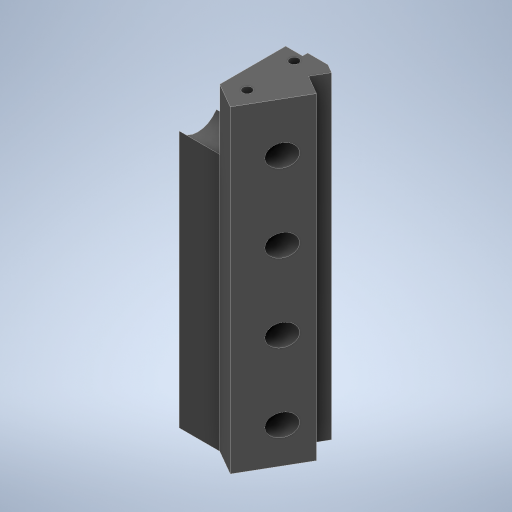
# Autodesk Inventor part: rail_base_outside
Saved by Autodesk Inventor 2024.1 (Build 281209000, 209)
## iProperties
Created: 2025-01-17
Part Number: rail_base_outside
Material: 一般
Document SubType Name: Modeling
Designer: hibik
Density: 1 g/cm^3
Appearance: 既定
Author: hibik
Autodesk Inventor part; units mm, degrees
sketch "スケッチ1" plane through (0, 0, 0) normal (0, 1, 0) x (-1, 0, 0)
  line L0 (0, 0) -> (-19.196896, -33.25)
  line L1 (0, 0) -> (30, 0) construction
  line L2 (30, 0) -> (30, -18)
  line L3 (30, -18) -> (18.452995, -38)
  line L4 (18.452995, -38) -> (-10.969655, -38)
  line L5 (-10.969655, -38) -> (-19.196896, -33.25)
  line L6 (30, -1.5) -> (-0.866025, -1.5)
  line L7 (25, -1.5) -> (5, -1.5)
  line L8 (5, -1.5) -> (5, -8)
  line L9 (5, -8) -> (25, -8) construction
  line L10 (25, -8) -> (25, -1.5)
  line L11 (30, -18) -> (21.919873, -13.334936)
  line L12 (21.919873, -13.334936) -> (25, -8)
  line L13 (30, -10.5) -> (25.669873, -8) construction
  line L14 (25.669873, -8) -> (22.422278, -13.625) construction
  line L15 (22.422278, -13.625) -> (26.752405, -16.125) construction
  line L16 (26.752405, -16.125) -> (30, -10.5) construction
  line L17 (5, -8) -> (12, -8)
  line L18 (12, -8) -> (12, -17)
  line L19 (12, -17) -> (5, -17)
  line L20 (5, -17) -> (5, -8) construction
  line L21 (5, -17) -> (0, -17)
  line L22 (0, -17) -> (-7.361216, -12.75)
  line L23 (0, -38) -> (0, -28)
  line L24 (0, -28) -> (24.226497, -28)
  line L25 (-13.567731, -36.5) -> (-11.067731, -32.169873)
  line L26 (-11.067731, -32.169873) -> (-16.696896, -28.919873)
  line L27 (0, -38) -> (-5, -38)
  line L28 (-5, -38) -> (-5, -36.5)
  line L29 (-5, -36.5) -> (0, -36.5)
  line L30 (0, -36.5) -> (0, -38)
  point P0 (-5, -38)
  point P1 (0, -36.5)
  dimension "d0" = 60
  dimension "d1" = 30
  dimension "d4" = 9.5
  dimension "d5" = 1.5
  dimension "d6" = 5
  dimension "d7" = 5
  dimension "d8" = 6.5
  dimension "d10" = 5
  dimension "d12" = 6.16025
  dimension "d14" = 9
  dimension "d15" = 7
  dimension "d18" = 10
  dimension "d19" = 10
  dimension "d20" = 6.5
  dimension "d21" = 5
  dimension "d22" = 3
  dimension "d23" = 5
  dimension "d24" = 1.5
  dimension "d26" = 38
  dimension "d27" = 18
  constraints: 62 end point, 11 parallel, 10 perpendicular, 10 point on line, 6 horizontal, 2 collinear, 2 vertical, 1 midpoint, 1 vertical alignment
  measures "d0" angle of L1 L0
  measures "d1" distance of L0.start L1.end
  measures "d4" distance from line of L4.end L0
  measures "d5" distance between parallel lines of L1 L6
  measures "d6" distance between parallel lines of L2 L10
  measures "d7" distance from line of L0.start L8
  measures "d8" distance of L9.end L7.start
  measures "d10" distance between parallel lines of L14 L16
  measures "d12" distance from line of L11 L9.end
  measures "d14" distance of L17.end L18.end
  measures "d15" distance of L18.end L19.end
  measures "d18" distance between parallel lines of L4 L24
  measures "d19" distance from line of L2.end L24
  measures "d20" distance between parallel lines of L0 L25
  measures "d21" distance between parallel lines of L5 L26
  measures "d22" distance from line of L4.end L25
  measures "d23" distance of L28.end L29.end
  measures "d24" distance of L27.end L28.end
  measures "d26" distance between parallel lines of L1 L4
  measures "d27" distance from line of L1 L2.end
extrude "押し出し1" add sketch "スケッチ1" along normal blind 94 contours L22 L21 L19 L18 L17 L8 L6 L10 L12 L11 L3 L24 L23 L29 L28 L4 L5 L25 L26 L0
sketch "スケッチ3" plane through (-12, 0, -8) normal (1, 0, 0) x (0, 0, -1)
  circle A0 centre (14.5, 79.5) radius 5.5
  line L0 (9, 0) -> (9, 94)
  line L1 (20, 0) -> (20, 94)
  line L2 (0, 94) -> (9, 94)
  line L3 (0, 94) -> (-6.5, 94)
  line L4 (-6.5, 94) -> (0, 94)
  line L5 (0, 94) -> (9, 94)
  line L6 (9, 94) -> (4.75, 94)
  line L7 (4.75, 94) -> (20.919873, 94)
  line L8 (20.919873, 94) -> (24.169873, 94)
  line L9 (24.169873, 94) -> (28.5, 94)
  line L10 (28.5, 94) -> (30, 94)
  line L11 (30, 94) -> (28.5, 94)
  line L12 (28.5, 94) -> (20, 94)
  line L13 (20, 94) -> (10, 94)
  line L14 (10, 94) -> (5.334936, 94)
  line L15 (5.334936, 94) -> (0, 94)
  circle A1 centre (14.5, 79.5) radius 6.5
  point P0 (-8, 0)
  point P1 (9, 79.5)
  point P2 (20, 79.5)
  point P3 (9, 82.964102)
  point P4 (20, 82.964102)
  dimension "d28" = 11
  dimension "d29" = 14.5
  dimension "d32" = 13
  constraints: 2 centre point, 2 tangent, 1 coincident
  measures "d28" diameter of A0
  measures "d29" distance from line of L2 A0.centre
  measures "d32" diameter of A1
extrude "押し出し2" cut sketch "スケッチ3" along normal up to surface (12 mm away)
sketch "スケッチ4" plane through (-12, 0, -8) normal (1, 0, 0) x (0, 0, -1)
  arc A0 (9, 76.035898) -> (20, 76.035898) centre (14.5, 79.5) ccw
  circle A1 centre (14.5, 79.5) radius 1.6
  point P0 (-8, 0)
  dimension "d33" = 3.2
  constraints: 1 centre point, 1 coincident
  measures "d33" diameter of A1
extrude "押し出し3" cut sketch "スケッチ4" against normal blind 8
sketch "スケッチ5" plane through (0, 0, -36.5) normal (-1, 0, 0) x (0, 0, 1)
  circle A0 centre (14, 79.5) radius 1.6 construction
  circle A1 centre (14, 79.5) radius 1.6
  line L0 (0, 0) -> (0, 94) projected
  circle A2 centre (14, 56.5) radius 1.6
  circle A3 centre (14, 33.5) radius 1.6
  circle A4 centre (14, 10.5) radius 1.6
  point P0 (36.5, 0)
  dimension "d36" = 3.2
  dimension "d39" = 23
  constraints: 4 centre point, 1 coincident, 1 vertical, 6 other
  measures "d36" diameter of A1
  measures "d39" distance of A1.centre A2.centre
extrude "押し出し4" cut sketch "スケッチ5" along normal through all both and the other way through all
ref_plane "作業平面1" through (-15, 0, -8) normal (1, 0, 0) x (0, 0, -1)
sketch "スケッチ6" plane through (-15, 0, -8) normal (1, 0, 0) x (0, 0, -1)
  circle A0 centre (14.5, 56.5) radius 1.6
  circle A1 centre (14.5, 33.5) radius 1.6
  circle A2 centre (14.5, 10.5) radius 1.6
  line L0 (17.790897, 79.5) -> (16.145448, 76.65)
  line L1 (16.145448, 76.65) -> (12.854552, 76.65)
  line L2 (12.854552, 76.65) -> (11.209103, 79.5)
  line L3 (11.209103, 79.5) -> (12.854552, 82.35)
  line L4 (12.854552, 82.35) -> (16.145448, 82.35)
  line L5 (16.145448, 82.35) -> (17.790897, 79.5)
  line L6 (17.790897, 56.5) -> (16.145448, 53.65)
  line L7 (16.145448, 53.65) -> (12.854552, 53.65)
  line L8 (12.854552, 53.65) -> (11.209103, 56.5)
  line L9 (11.209103, 56.5) -> (12.854552, 59.35)
  line L10 (12.854552, 59.35) -> (16.145448, 59.35)
  line L11 (16.145448, 59.35) -> (17.790897, 56.5)
  line L12 (17.790897, 33.5) -> (16.145448, 30.65)
  line L13 (16.145448, 30.65) -> (12.854552, 30.65)
  line L14 (12.854552, 30.65) -> (11.209103, 33.5)
  line L15 (11.209103, 33.5) -> (12.854552, 36.35)
  line L16 (12.854552, 36.35) -> (16.145448, 36.35)
  line L17 (16.145448, 36.35) -> (17.790897, 33.5)
  line L18 (17.790897, 10.5) -> (16.145448, 7.65)
  line L19 (16.145448, 7.65) -> (12.854552, 7.65)
  line L20 (12.854552, 7.65) -> (11.209103, 10.5)
  line L21 (11.209103, 10.5) -> (12.854552, 13.35)
  line L22 (12.854552, 13.35) -> (16.145448, 13.35)
  line L23 (16.145448, 13.35) -> (17.790897, 10.5)
  circle A3 centre (14.5, 79.5) radius 1.6
  point P0 (-8, 0)
  dimension "d47" = 5.7
  constraints: 48 end point, 4 coincident, 4 horizontal, 3 parallel, 52 other
  measures "d47" distance between parallel lines of L1 L4
extrude "押し出し5" cut sketch "スケッチ6" against normal through all contours A0 | A1 | A2 | L0 L1 L2 L3 L4 L5 | L6 L7 L8 L9 L10 L11 | L12 L13 L14 L15 L16 L17 | L18 L19 L20 L21 L22 L23 | A3
ref_plane "作業平面2" through (2, 0, -36.5) normal (-1, 0, 0) x (0, 0, 1)
sketch "スケッチ7" plane through (2, 0, -36.5) normal (-1, 0, 0) x (0, 0, 1)
  circle A0 centre (14, 79.5) radius 1.6 projected
  circle A1 centre (14, 56.5) radius 1.6 projected
  circle A2 centre (14, 33.5) radius 1.6 projected
  circle A3 centre (14, 10.5) radius 1.6 projected
  circle A4 centre (14, 79.5) radius 3.25
  circle A5 centre (14, 56.5) radius 1.6 projected
  circle A6 centre (14, 56.5) radius 3.25
  circle A7 centre (14, 33.5) radius 3.25
  circle A8 centre (14, 10.5) radius 3.25
  point P0 (36.5, 0)
  dimension "d51" = 6.5
  dimension "d52" = 6.5
  dimension "d53" = 6.5
  dimension "d54" = 6.5
  constraints: 4 centre point, 4 coincident
  measures "d51" diameter of A4
  measures "d52" diameter of A6
  measures "d53" diameter of A7
  measures "d54" diameter of A8
extrude "押し出し6" cut sketch "スケッチ7" against normal through all contours A0 | A1 | A2 | A3 | A4 | A6 | A7 | A8
sketch "スケッチ8" plane through (-25, 0, -1.5) normal (0, 0, 1) x (1, 0, 0)
  circle A0 centre (5, 77) radius 1.6 construction
  circle A1 centre (15, 77) radius 1.6 construction
  circle A2 centre (5, 47) radius 1.6 construction
  circle A3 centre (15, 47) radius 1.6 construction
  circle A4 centre (5, 17) radius 1.6 construction
  circle A5 centre (15, 17) radius 1.6 construction
  circle A6 centre (5, 77) radius 1.35
  circle A7 centre (15, 77) radius 1.35
  circle A8 centre (5, 47) radius 1.35
  circle A9 centre (15, 47) radius 1.35
  circle A10 centre (5, 17) radius 1.35
  circle A11 centre (15, 17) radius 1.35
  point P0 (25, 0)
  dimension "d59" = 2.7
  constraints: 6 centre point, 6 coincident, 5 equal radius
  measures "d59" diameter of A6
extrude "押し出し7" cut sketch "スケッチ8" against normal blind 5
ref_plane "作業平面3" through (0, 7, 0) normal (0, -1, 0) x (1, 0, 0)
sketch "スケッチ9" plane through (0, 7, 0) normal (0, -1, 0) x (1, 0, 0)
  line L0 (0, -38) -> (10.1, -38)
  line L1 (10.1, -38) -> (10.1, -30.8)
  line L2 (10.1, -30.8) -> (0, -30.8)
  line L3 (0, -30.8) -> (0, -38)
  line L4 (10.969655, -38) -> (-1, -38)
  point P0 (0, 0)
  point P1 (0, -36.5)
  dimension "d61" = 10.1
  dimension "d62" = 7.2
  constraints: 8 end point, 2 parallel, 1 collinear, 1 horizontal, 1 perpendicular, 1 point on line
  measures "d61" distance of L2.end L1.end
  measures "d62" distance of L1.end L0.end
extrude "押し出し8" cut sketch "スケッチ9" against normal blind 7.2
sketch "スケッチ11" plane through (0, 7, 0) normal (0, 1, 0) x (1, 0, 0)
  line L0 (5, 36.5) -> (5, 38) projected
  line L1 (5, 38) -> (0, 38)
  line L2 (0, 38) -> (0, 36.5)
  line L3 (0, 36.5) -> (5, 36.5)
  line L4 (5, 36.5) -> (5, 38)
  point P0 (0, 0)
  constraints: 8 end point, 2 parallel, 1 horizontal, 1 perpendicular
extrude "押し出し9" add sketch "スケッチ11" against normal up to surface (7 mm away)
sketch "スケッチ12" plane through (0, 14.2, 0) normal (0, -1, 0) x (1, 0, 0)
  line L0 (5, -36.5) -> (0, -36.5) projected
  line L1 (5, -38) -> (0, -38)
  line L2 (0, -38) -> (0, -36.5)
  line L3 (0, -36.5) -> (5, -36.5)
  line L4 (5, -36.5) -> (5, -38)
  point P0 (0, 0)
  constraints: 8 end point, 2 parallel, 1 horizontal, 1 perpendicular
extrude "押し出し10" add sketch "スケッチ12" against normal blind 10
sketch "スケッチ14" plane through (0, 0, 0) normal (0, -1, 0) x (1, 0, 0)
  circle A0 centre (5, -34) radius 1.6 projected
  point P0 (0, 0)
extrude "押し出し11" cut sketch "スケッチ14" against normal blind 30
sketch "スケッチ15" plane through (0, 0, 0) normal (0, -1, 0) x (1, 0, 0)
  circle A0 centre (5, -34) radius 1.6 projected
  circle A1 centre (5, -34) radius 2.5
  point P0 (0, 0)
  dimension "d71" = 5
  constraints: 1 centre point, 1 coincident
  measures "d71" diameter of A1
extrude "押し出し12" cut sketch "スケッチ15" against normal blind 4 contours A0 | A1
sketch "スケッチ16" plane through (0, 24.2, 0) normal (0, 1, 0) x (1, 0, 0)
  circle A0 centre (5, 34) radius 1.6
  line L0 (3.354552, 36.85) -> (6.645448, 36.85)
  line L1 (6.645448, 36.85) -> (8.290897, 34)
  line L2 (8.290897, 34) -> (6.645448, 31.15)
  line L3 (6.645448, 31.15) -> (3.354552, 31.15)
  line L4 (3.354552, 31.15) -> (1.709103, 34)
  line L5 (1.709103, 34) -> (3.354552, 36.85)
  line L6 (8.290897, 34) -> (8.290897, 38)
  line L7 (1.709103, 34) -> (1.709103, 38)
  line L8 (8.290897, 38) -> (1.709103, 38)
  line L9 (5, 38) -> (0, 38)
  point P0 (0, 0)
  dimension "d74" = 5.7
  constraints: 18 end point, 2 horizontal, 2 vertical, 1 coincident, 1 collinear, 13 other
  measures "d74" distance between parallel lines of L3 L0
extrude "押し出し13" cut sketch "スケッチ16" against normal blind 4 contours A0 | L5 L7 L8 L6 L1 L0 | L0 L1 L2 L3 L4 L5
ref_plane "作業平面4" through (0, 14, 0) normal (0, -1, 0) x (1, 0, 0)
sketch "スケッチ17" plane through (0, 14, 0) normal (0, -1, 0) x (1, 0, 0)
  line L0 (-28.351924, -20.854552) -> (-29.301924, -19.209103)
  line L1 (-29.301924, -19.209103) -> (-28.351924, -20.854552)
  line L2 (-28.351924, -20.854552) -> (-26.451924, -24.145448)
  line L3 (-26.451924, -24.145448) -> (-25.501924, -25.790897)
  line L4 (-25.501924, -25.790897) -> (-26.451924, -24.145448)
  line L5 (-26.451924, -24.145448) -> (-28.351924, -20.854552)
  line L6 (-28.351924, -20.854552) -> (-29.301924, -19.209103)
  line L7 (-29.301924, -19.209103) -> (-28.351924, -20.854552)
  line L8 (-28.351924, -20.854552) -> (-26.451924, -24.145448)
  line L9 (-26.451924, -24.145448) -> (-25.501924, -25.790897)
  line L10 (-25.501924, -25.790897) -> (-26.451924, -24.145448)
  line L11 (-26.451924, -24.145448) -> (-28.351924, -20.854552)
  line L12 (-28.351924, -20.854552) -> (-29.301924, -19.209103)
  line L13 (-29.301924, -19.209103) -> (-28.351924, -20.854552)
  line L14 (-28.351924, -20.854552) -> (-26.451924, -24.145448)
  line L15 (-26.451924, -24.145448) -> (-25.501924, -25.790897)
  line L16 (-25.501924, -25.790897) -> (-26.451924, -24.145448)
  line L17 (-26.451924, -24.145448) -> (-28.351924, -20.854552)
  line L18 (-28.351924, -20.854552) -> (-29.301924, -19.209103)
  line L19 (-29.301924, -19.209103) -> (-28.351924, -20.854552)
  line L20 (-28.351924, -20.854552) -> (-26.451924, -24.145448)
  line L21 (-26.451924, -24.145448) -> (-25.501924, -25.790897)
  line L22 (-25.501924, -25.790897) -> (-26.451924, -24.145448)
  line L23 (-26.451924, -24.145448) -> (-28.351924, -20.854552)
  line L24 (-24.226497, -28) -> (-30, -18)
  line L25 (-24.226497, -28) -> (-30, -18)
  line L26 (-26.330127, -34.356406) -> (-31.526279, -37.356406)
  line L27 (-31.526279, -37.356406) -> (-39.026279, -24.366025)
  line L28 (-39.026279, -24.366025) -> (-33.830127, -21.366025)
  line L29 (-33.830127, -21.366025) -> (-26.330127, -34.356406)
  line L30 (-24.226497, -28) -> (-26.330127, -34.356406)
  line L31 (-33.830127, -21.366025) -> (-29.5, -18.866025)
  point P0 (0, 0)
  dimension "d78" = 1
  dimension "d79" = 15
  dimension "d80" = 11
  dimension "d81" = 6
  constraints: 12 end point, 3 parallel, 2 point on line, 1 perpendicular
  measures "d78" distance from line of L24.end L28
  measures "d79" distance between parallel lines of L26 L28
  measures "d80" distance between parallel lines of L24 L27
  measures "d81" distance between parallel lines of L27 L29
extrude "押し出し14" add sketch "スケッチ17" against normal blind 2
fillet "フィレット1" radius 3 1 edges at (-26.8632, 16, -23.433)
sketch "スケッチ18" plane through (5, 94, -36.5) normal (0, 0, -1) x (-1, 0, 0)
  circle A0 centre (2.5, -10) radius 1.6 projected
  circle A1 centre (2.5, -35) radius 1.6 projected
  circle A2 centre (2.5, -60) radius 1.6 projected
  circle A3 centre (2.5, -10) radius 1.35
  circle A4 centre (2.5, -35) radius 1.35
  circle A5 centre (2.5, -60) radius 1.35
  point P0 (5, -94)
  dimension "d85" = 2.7
  constraints: 3 centre point, 3 coincident, 2 equal radius
  measures "d85" diameter of A3
extrude "押し出し15" cut sketch "スケッチ18" against normal blind 5 contours A3 | A4 | A5
sketch "スケッチ19" plane through (0, 94, 0) normal (0, 1, 0) x (1, 0, 0)
  line L0 (2, 25.75) -> (14.866769, 25.75)
  circle A0 centre (5, 34) radius 1.6
  circle A1 centre (5.531089, 19.580127) radius 1.6
  circle A2 centre (-16, 8) radius 1.6
  circle A3 centre (-22.535898, 22.928203) radius 1.6
  line L1 (19.196896, 33.25) -> (10.969655, 38)
  line L2 (10.969655, 38) -> (10.969655, 39)
  line L3 (10.969655, 39) -> (-18.452995, 39)
  line L4 (-18.452995, 39) -> (-18.452995, 38)
  line L5 (-18.452995, 38) -> (-30, 18)
  line L6 (-30, 1.5) -> (0.866025, 1.5)
  line L7 (0.866025, 1.5) -> (19.196896, 33.25)
  circle A4 centre (5, 34) radius 1.35
  circle A5 centre (5.531089, 19.580127) radius 1.35
  circle A6 centre (-22.535898, 22.928203) radius 1.35
  circle A7 centre (-16, 8) radius 1.35
  line L8 (-30, 18) -> (-30, 1.5)
  point P0 (0, 0)
  dimension "d88" = 2.7
  dimension "d89" = 2.7
  dimension "d90" = 2.7
  dimension "d91" = 2.7
  constraints: 4 centre point, 4 coincident
  measures "d88" diameter of A4
  measures "d89" diameter of A5
  measures "d90" diameter of A6
  measures "d91" diameter of A7
extrude "押し出し16" cut sketch "スケッチ19" against normal blind 10 contours A4 | A5 | A6 | A7
ref_plane "作業平面5" through (0, 47, 0) normal (0, 1, 0) x (1, 0, 0)
mirror "ミラー1" about plane through (0, 47, 0) normal (0, 1, 0) of "押し出し16"
sketch "スケッチ20" plane through (0, 0, 0) normal (0, -1, 0) x (1, 0, 0)
  circle A0 centre (-6, -23) radius 1.35
  line L0 (0, -28) -> (-24.226497, -28)
  point P0 (0, 0)
  dimension "d95" = 2.7
  dimension "d96" = 5
  dimension "d97" = 6
  constraints: 1 centre point
  measures "d95" diameter of A0
  measures "d96" distance from line of L0 A0.centre
  measures "d97" horizontal distance of L0.start A0.centre
extrude "押し出し17" cut sketch "スケッチ20" against normal blind 10
ref_plane "作業平面6" through (-18, 0, -8) normal (-1, 0, 0) x (0, 0, 1)
sketch "スケッチ22" plane through (-18, 0, -8) normal (-1, 0, 0) x (0, 0, 1)
  circle A0 centre (-14.5, 79.5) radius 1.6
  line L0 (-16.145448, 82.35) -> (-12.854552, 82.35)
  line L1 (-17.790897, 79.5) -> (-16.145448, 82.35)
  line L2 (-16.145448, 76.65) -> (-17.790897, 79.5)
  line L3 (-12.854552, 76.65) -> (-16.145448, 76.65)
  line L4 (-11.209103, 79.5) -> (-12.854552, 76.65)
  line L5 (-12.854552, 82.35) -> (-11.209103, 79.5)
  circle A1 centre (-14.5, 56.5) radius 1.6
  line L6 (-16.145448, 59.35) -> (-12.854552, 59.35)
  line L7 (-17.790897, 56.5) -> (-16.145448, 59.35)
  line L8 (-16.145448, 53.65) -> (-17.790897, 56.5)
  line L9 (-12.854552, 53.65) -> (-16.145448, 53.65)
  line L10 (-11.209103, 56.5) -> (-12.854552, 53.65)
  line L11 (-12.854552, 59.35) -> (-11.209103, 56.5)
  circle A2 centre (-14.5, 33.5) radius 1.6
  line L12 (-16.145448, 36.35) -> (-12.854552, 36.35)
  line L13 (-17.790897, 33.5) -> (-16.145448, 36.35)
  line L14 (-16.145448, 30.65) -> (-17.790897, 33.5)
  line L15 (-12.854552, 30.65) -> (-16.145448, 30.65)
  line L16 (-11.209103, 33.5) -> (-12.854552, 30.65)
  line L17 (-12.854552, 36.35) -> (-11.209103, 33.5)
  circle A3 centre (-14.5, 10.5) radius 1.6
  line L18 (-16.145448, 13.35) -> (-12.854552, 13.35)
  line L19 (-17.790897, 10.5) -> (-16.145448, 13.35)
  line L20 (-16.145448, 7.65) -> (-17.790897, 10.5)
  line L21 (-12.854552, 7.65) -> (-16.145448, 7.65)
  line L22 (-11.209103, 10.5) -> (-12.854552, 7.65)
  line L23 (-12.854552, 13.35) -> (-11.209103, 10.5)
  line L24 (-10.747223, 10.5) -> (-12.623612, 7.25)
  line L25 (-12.623612, 7.25) -> (-16.376388, 7.25)
  line L26 (-16.376388, 7.25) -> (-18.252777, 10.5)
  line L27 (-18.252777, 10.5) -> (-16.376388, 13.75)
  line L28 (-16.376388, 13.75) -> (-12.623612, 13.75)
  line L29 (-12.623612, 13.75) -> (-10.747223, 10.5)
  line L30 (-10.747223, 33.5) -> (-12.623612, 30.25)
  line L31 (-12.623612, 30.25) -> (-16.376388, 30.25)
  line L32 (-16.376388, 30.25) -> (-18.252777, 33.5)
  line L33 (-18.252777, 33.5) -> (-16.376388, 36.75)
  line L34 (-16.376388, 36.75) -> (-12.623612, 36.75)
  line L35 (-12.623612, 36.75) -> (-10.747223, 33.5)
  line L36 (-10.747223, 79.5) -> (-12.623612, 76.25)
  line L37 (-12.623612, 76.25) -> (-16.376388, 76.25)
  line L38 (-16.376388, 76.25) -> (-18.252777, 79.5)
  line L39 (-18.252777, 79.5) -> (-16.376388, 82.75)
  line L40 (-16.376388, 82.75) -> (-12.623612, 82.75)
  line L41 (-12.623612, 82.75) -> (-10.747223, 79.5)
  line L42 (-10.747223, 56.5) -> (-12.623612, 53.25)
  line L43 (-12.623612, 53.25) -> (-16.376388, 53.25)
  line L44 (-16.376388, 53.25) -> (-18.252777, 56.5)
  line L45 (-18.252777, 56.5) -> (-16.376388, 59.75)
  line L46 (-16.376388, 59.75) -> (-12.623612, 59.75)
  line L47 (-12.623612, 59.75) -> (-10.747223, 56.5)
  point P0 (8, 0)
  dimension "d101" = 6.5
  constraints: 48 end point, 4 coincident, 4 horizontal, 3 parallel, 52 other
  measures "d101" distance between parallel lines of L37 L40
extrude "押し出し18" cut sketch "スケッチ22" along normal through all contours A0 | L0 L5 L4 L3 L2 L1 | A1 | L6 L11 L10 L9 L8 L7 | A2 | L12 L17 L16 L15 L14 L13 | A3 | L18 L23 L22 L21 L20 L19 | L24 L25 L26 L27 L28 L29 | L30 L31 L32 L33 L34 L35 | L36 L37 L38 L39 L40 L41 | L42 L43 L44 L45 L46 L47
sketch "スケッチ23" plane through (-12, 0, -8) normal (1, 0, 0) x (0, 0, -1)
  circle A0 centre (14.5, 79.5) radius 1.6
  line L0 (0, 94) -> (20, 94)
  line L1 (0, 0) -> (0, 94)
  line L2 (0, 0) -> (9, 0)
  line L3 (9, 0) -> (9, 76.035898)
  arc A1 (9, 76.035898) -> (20, 76.035898) centre (14.5, 79.5) ccw
  line L4 (20, 94) -> (20, 76.035898)
  line L5 (0, 94) -> (141.423362, 94)
  line L6 (141.423362, 94) -> (141.423362, -78.894064)
  line L7 (141.423362, -78.894064) -> (0, -78.894064)
  line L8 (0, -78.894064) -> (0, 94)
  line L9 (4.5, 94) -> (-67.595329, 94)
  line L10 (-67.595329, 94) -> (-67.595329, -75.008048)
  line L11 (-67.595329, -75.008048) -> (4.5, -75.008048)
  line L12 (4.5, -75.008048) -> (4.5, 94)
  point P0 (-8, 0)
  point P1 (0, -75.008048)
  point P2 (4.5, 0)
  constraints: 16 end point, 4 parallel, 2 horizontal, 2 perpendicular, 1 point on line
extrude "押し出し19" cut sketch "スケッチ23" against normal through all contours L0 L12 L2 L1 | L1 L8 L11 L10 L9 | L0 L4 A1 L3 L2 L12 | L5 L6 L7 L8 L11 L12 L2 L3 A1 L4
sketch "スケッチ24" plane through (-12, 0, -8) normal (-1, 0, 0) x (0, 0, 1)
  line L0 (-2.174773, 100.003485) -> (52.478296, 100.003485)
  line L1 (52.478296, 100.003485) -> (52.478296, -68.607042)
  line L2 (52.478296, -68.607042) -> (-2.174773, -68.607042)
  line L3 (-2.174773, -68.607042) -> (-2.174773, 100.003485)
  point P0 (8, 0)
  constraints: 8 end point, 2 parallel, 1 horizontal, 1 perpendicular
extrude "押し出し20" cut sketch "スケッチ24" against normal through all
equation "\"d52\" = d51"
equation "\"d53\" = d52"
equation "\"d54\" = d53"
